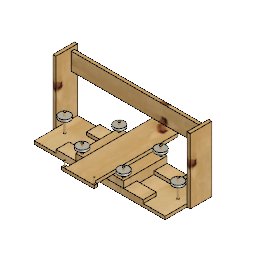
model_X v5 (Autodesk Fusion 360 design; units mm, degrees)
Autodesk Fusion 360 part; units mm, degrees
sketch "p1" plane through (0, 0, 0) normal (0, 0, 1) x (1, 0, 0)
  line L0 (300, 100) -> (-300, 100)
  line L1 (-300, 100) -> (-300, -100)
  line L2 (-300, -100) -> (300, -100)
  line L3 (300, -100) -> (300, 100)
  line L4 (300, 100) -> (-300, -100) construction
  line L5 (-300, 100) -> (300, -100) construction
  circle A0 centre (-260, 0) radius 5
  circle A1 centre (260, 0) radius 5
  line L6 (-200, -100) -> (200, -100)
  line L7 (200, -100) -> (200, -40)
  line L8 (200, -40) -> (-200, -40)
  line L9 (-200, -40) -> (-200, -100)
  line L10 (-200, 100) -> (200, 100)
  line L11 (200, 100) -> (200, 40)
  line L12 (200, 40) -> (-200, 40)
  line L13 (-200, 40) -> (-200, 100)
  circle A2 through (-235, 0, 75) (-272.5, 21.6506, 75) (-272.5, -21.6506, 75)
  circle A3 through (285, 0, 75) (247.5, 21.6506, 75) (247.5, -21.6506, 75)
  dimension "d1" = 600
  dimension "d2" = 200
  dimension "d3" = 40
  dimension "d4" = 40
  dimension "d5" = 10
  dimension "d6" = 10
  dimension "d7" = 400
  dimension "d8" = 60
  dimension "d9" = 400
  dimension "d10" = 60
  dimension "d11" = 100
  dimension "d12" = 100
  measures "d5" diameter of A0
  measures "d6" diameter of A1
  measures "d9" distance of L11 L13
  measures "d10" distance of L0 L12
  measures "d12" distance of L3 L7
extrude "Extrude1" add sketch "p1" along normal blind 15 contours L0 L1 L2 L3 L7 L8 L9 L11 L12 L13 | L0 L10 L11 L12 L13 | L2 L6 L7 L8 L9 | A0 | A1 makes body 1
extrude "Extrude2" add sketch "p1" along normal blind 30 contours L0 L10 L11 L12 L13 | L2 L6 L7 L8 L9 bodies 1
extrude "Extrude3" add sketch "p1" along normal blind 100 contours A0 | A1 bodies 1
ref_plane "WorkPlane1" through (0, 0, 30) normal (0, 0, 1) x (1, 0, 0)
sketch "p2" plane through (0, 0, 30) normal (0, 0, 1) x (1, 0, 0)
  line L0 (110, 39.5) -> (-110, 39.5)
  line L1 (-110, 39.5) -> (-110, -39.5)
  line L2 (-110, -39.5) -> (110, -39.5)
  line L3 (110, -39.5) -> (110, 39.5)
  line L4 (110, 39.5) -> (-110, -39.5) construction
  line L5 (-110, 39.5) -> (110, -39.5) construction
  line L6 (-110, 100) -> (110, 100)
  line L7 (110, 100) -> (110, -100)
  line L8 (110, -100) -> (-110, -100)
  line L9 (-110, -100) -> (-110, 100)
  line L10 (300, 100) -> (-300, 100)
  line L11 (-300, -100) -> (300, -100)
  circle A0 centre (-95, -85) radius 5
  circle A1 centre (95, -85) radius 5
  circle A2 centre (-95, 85) radius 5
  circle A3 centre (95, 85) radius 5
  circle A4 through (120, -85, 50) (82.5, -63.3494, 50) (82.5, -106.6506, 50)
  circle A5 through (-70, -85, 50) (-107.5, -63.3494, 50) (-107.5, -106.6506, 50)
  circle A6 through (-70, 85, 50) (-107.5, 106.6506, 50) (-107.5, 63.3494, 50)
  circle A7 through (120, 85, 50) (82.5, 106.6506, 50) (82.5, 63.3494, 50)
  line L12 (-70, -85) -> (-70, -100) construction
  line L13 (69.9377, -85) -> (70, -100) construction
  line L14 (70, 85) -> (70, 100) construction
  line L15 (-70, 85) -> (-70, 100) construction
  line L16 (70, -100) -> (60, -100) construction
  line L17 (-70, 100) -> (-60, 100) construction
  line L18 (-60, 100) -> (60, 100)
  line L19 (60, 100) -> (60, -100)
  line L20 (60, -100) -> (-60, -100)
  line L21 (-60, -100) -> (-60, 100)
  line L22 (30, 100) -> (-30, 100)
  line L23 (-30, 100) -> (-30, -100)
  line L24 (-30, -100) -> (30, -100)
  line L25 (30, -100) -> (30, 100)
  line L26 (30, 100) -> (-30, -100) construction
  line L27 (-30, 100) -> (30, -100) construction
  dimension "d20" = 220
  dimension "d21" = 79
  dimension "d22" = 220
  dimension "d27" = 10
  dimension "d28" = 15
  dimension "d29" = 15
  dimension "d30" = 10
  dimension "d31" = 10
  dimension "d32" = 10
  dimension "d33" = 15
  dimension "d34" = 15
  dimension "d35" = 15
  dimension "d36" = 15
  dimension "d37" = 15
  dimension "d38" = 15
  dimension "d59" = 10
  dimension "d60" = 10
  dimension "d61" = 120
  dimension "d62" = 200
  dimension "d63" = 60
  measures "d22" distance of L7 L9
  measures "d27" diameter of A0
  measures "d30" diameter of A1
  measures "d31" diameter of A2
  measures "d32" diameter of A3
extrude "Extrude6" add sketch "p2" against normal blind 14 separate body contours L0 L2 L3 L7 L19 | L0 L2 L19 L25 | L0 L2 L23 L25 | L0 L2 L21 L23 | L0 L1 L2 L9 L21 makes body 2
sketch "p1 (curves 75 mm off its plane)" plane through (0, 0, 75) normal (0, 0, 1) x (1, 0, 0)
  circle A0 centre (-260, 0) radius 25
  circle A1 centre (260, 0) radius 25
extrude "Extrude4" add sketch "p1 (curves 75 mm off its plane)" along normal blind 10 separate body makes body 3 at (-264.7538, 2.2158, 75) makes body 4 at (265.8316, 4.4538, 75)
extrude "Extrude7" add sketch "p2" along normal blind 15 contours L0 L2 L3 L7 L19 | L0 L6 L7 L10 L19 | L0 L2 L19 L25 | L0 L6 L10 L18 L19 L25 | L2 L7 L8 L11 L19 | L0 L2 L23 L25 | L0 L6 L10 L18 L22 L23 L25 | L2 L8 L11 L19 L20 L25 | L0 L2 L21 L23 | L0 L6 L10 L18 L21 L23 | L2 L8 L11 L20 L23 L24 L25 | L0 L1 L2 L9 L21 | L0 L6 L9 L10 L21 | L2 L8 L11 L20 L21 L23 | L2 L8 L9 L11 L21 | A0 | A1 | A2 | A3 bodies 2
extrude "Extrude8" add sketch "p2" along normal blind 70 contours A0 | A1 | A2 | A3 bodies 2
sketch "p2 (curves 50 mm off its plane)" plane through (0, 0, 80) normal (0, 0, 1) x (1, 0, 0)
  circle A0 centre (95, -85) radius 25
  circle A1 centre (-95, -85) radius 25
  circle A2 centre (-95, 85) radius 25
  circle A3 centre (95, 85) radius 25
extrude "Extrude9" add sketch "p2 (curves 50 mm off its plane)" along normal blind 10 separate body makes body 5 at (92.4105, -86.6853, 80) makes body 6 at (88.6141, 88.0753, 80) makes body 7 at (-97.5895, -86.6853, 80) makes body 8 at (-101.3859, 88.0753, 80)
extrude "Extrude10" add sketch "p2" along normal blind 30 contours L0 L2 L3 L7 L19 | L0 L6 L7 L10 L19 | L0 L2 L19 L25 | L0 L6 L10 L18 L19 L25 | L2 L7 L8 L11 L19 | L2 L8 L11 L19 L20 L25 | L0 L2 L21 L23 | L0 L6 L10 L18 L21 L23 | L0 L1 L2 L9 L21 | L0 L6 L9 L10 L21 | L2 L8 L11 L20 L21 L23 | L2 L8 L9 L11 L21 bodies 2
ref_plane "WorkPlane2" through (0, 0, 60) normal (0, 0, 1) x (1, 0, 0)
sketch "p3" plane through (0, 0, 60) normal (0, 0, 1) x (1, 0, 0)
  line L0 (-30, -100) -> (30, -100)
  line L1 (30, -100) -> (30, 100)
  line L2 (30, 100) -> (-30, 100)
  line L3 (-30, 100) -> (-30, -100)
  line L4 (60, 200) -> (-60, 200)
  line L5 (-60, 200) -> (-60, -200)
  line L6 (-60, -200) -> (60, -200)
  line L7 (60, -200) -> (60, 200)
  line L8 (60, 200) -> (-60, -200) construction
  line L9 (-60, 200) -> (60, -200) construction
  line L10 (60, -200) -> (75, -200)
  line L11 (75, -200) -> (75, -185)
  line L12 (75, -185) -> (60, -185)
  line L13 (60, -185) -> (60, -200)
  line L14 (-60, -200) -> (-75, -200)
  line L15 (-75, -200) -> (-75, -185)
  line L16 (-75, -185) -> (-60, -185)
  line L17 (-60, -185) -> (-60, -200)
  line L18 (-60, 200) -> (-75, 200)
  line L19 (-60, 185) -> (-60, 200)
  line L20 (60, 185) -> (60, 200)
  line L21 (10, 255) -> (-5, 255)
  line L22 (0, 200) -> (7.5, 200)
  line L23 (7.5, 200) -> (7.5, 240)
  line L24 (7.5, 240) -> (-7.5, 240)
  line L25 (-7.5, 240) -> (-7.5, 200)
  line L26 (7.5, 200) -> (-7.5, 200)
  circle A0 centre (0, 234.9202) radius 5
  circle A1 through (25, 234.9202, 20) (-12.5, 256.5708, 20) (-12.5, 213.2695, 20)
  circle A2 centre (-95, -85) radius 25 construction
  circle A3 centre (95, -85) radius 25 construction
  line L27 (-95, -110) -> (95, -110) construction
  line L28 (60, -100) -> (-60, -100) construction
  line L29 (-95, 110) -> (95, 110) construction
  circle A4 centre (67.5, -192.5) radius 2.5
  circle A5 centre (-67.5, -192.5) radius 2.5
  dimension "d67" = 400
  dimension "d72" = 15
  dimension "d73" = 15
  dimension "d74" = 15
  dimension "d75" = 15
  dimension "d82" = 7.5
  dimension "d83" = 40
  dimension "d84" = 15
  dimension "d87" = 10
  dimension "d93" = 220
  dimension "d94" = 90
  dimension "d95" = 90
  dimension "d96" = 5
  dimension "d97" = 5
  measures "d82" distance of origin
  measures "d87" diameter of A0
  measures "d94" distance of L4 L29
  measures "d95" distance of L10 L27
  measures "d96" diameter of A4
  measures "d97" diameter of A5
extrude "Extrude11" add sketch "p3" against normal blind 14 separate body contours L0 L1 L2 L3 makes body 9
extrude "Extrude12" add sketch "p3" along normal blind 15 contours L0 L1 L2 L3 | L4 L5 L6 L7 L13 L17 L19 L20 L22 L26 bodies 9
extrude "Extrude13" add sketch "p3" along normal blind 15 contours L4 L22 L23 L24 L25 L26 | L7 L10 L11 L12 L13 | L5 L14 L15 L16 L17 | A0 | A4 | A5 bodies 9
extrude "Extrude14" add sketch "p3" along normal blind 40 contours A0 bodies 9
sketch "p3 (curves 20 mm off its plane)" plane through (0, 0, 80) normal (0, 0, 1) x (1, 0, 0)
  circle A0 centre (0, 234.9202) radius 25
extrude "Extrude15" add sketch "p3 (curves 20 mm off its plane)" along normal blind 10 separate body makes body 10
copy_body "Body->Comp1" bodies 1 removing the originals makes body 11 in component "Component"
copy_body "Body->Comp2" bodies 2 removing the originals makes body 12 in component "Component'"
copy_body "Body->Comp3" bodies 9 removing the originals makes body 13 in component "Component''"
copy_body "CutPasteBodies1" bodies 10 removing the originals makes body 14 in component "Component''"
copy_body "CutPasteBodies1'" bodies 5 7 6 8 removing the originals makes body 15 makes body 16 makes body 17 makes body 18 in component "Component'"
copy_body "CutPasteBodies1''" bodies 4 3 removing the originals makes body 19 makes body 20 in component "Component"
extrude "Extrude1'" add sketch "p3" along normal blind 40 contours A4 | A5 bodies 13 in component "Component''"
sketch "linha" plane through (0.0019, 0.0411, 85) normal (0, 0, 1) x (-1, 0, 0)
  circle A0 centre (-259.9981, 0.0411) radius 25
  line L0 (-74.9981, 185.0411) -> (-59.9981, 185.0411)
  line L1 (-67.4981, 185.0411) -> (-69.9357, 85.0411)
  circle A1 centre (-94.9981, 85.0411) radius 25
  line L2 (-92.9821, 60.1225) -> (-261.4996, 24.996)
  circle A2 centre (-94.9981, -84.9589) radius 25
  line L3 (-262.0665, -24.8732) -> (-89.9342, -60.4771)
  circle A3 centre (0.0019, -234.8791) radius 25
  line L4 (-70.1205, -82.4879) -> (-59.9981, -199.9589)
  line L5 (-59.9981, -199.9589) -> (-20.3331, -249.4217)
  line L6 (22.409, -245.966) -> (60.0019, -199.9589)
  line L7 (60.0019, -199.9589) -> (70.0019, -84.9589)
  circle A4 centre (260.0019, 0.0411) radius 25
  circle A5 centre (95.0019, -84.9589) radius 25
  line L8 (260.8771, -24.9436) -> (89.9139, -60.4821)
  circle A6 centre (95.0019, 85.0411) radius 25
  line L9 (264.1198, 24.6996) -> (89.9608, 60.5546)
  line L10 (75.0019, 185.0411) -> (60.0019, 185.0411)
  line L11 (67.5019, 185.0411) -> (70.0019, 85.0411)
  arc A7 (70.0019, 85.0411) -> (89.9608, 60.5546) centre (95.0019, 85.0411) ccw
  arc A8 (-92.9821, 60.1225) -> (-69.9357, 85.0411) centre (-95.0512, 85.1528) ccw
  arc A9 (-261.4996, 24.996) -> (-262.0665, -24.8732) centre (-259.9981, 0.0411) ccw
  arc A10 (-69.9981, -84.9589) -> (-89.9342, -60.4771) centre (-94.9981, -84.9589) ccw
  arc A11 (-20.3331, -249.4217) -> (22.409, -245.966) centre (0.0019, -234.8791) ccw
  arc A12 (89.9139, -60.4821) -> (70.0019, -84.9589) centre (91.4397, -82.061) ccw
  arc A13 (260.8771, -24.9436) -> (264.1198, 24.6996) centre (260.0019, 0.0411) ccw
  line L12 (-67.4981, 185.0411) -> (-67.4981, 192)
  line L13 (67.5019, 185.0411) -> (67.5019, 190.4198)
  line L14 (67.5019, 190.4198) -> (67.5019, 192)
sketch "Sketch5" plane through (0, 0, 0) normal (0, 0, 1) x (1, 0, 0)
  line L0 (300, 0) -> (315, 0)
  line L1 (315, 0) -> (315, 100)
  line L2 (315, 100) -> (300, 100)
  line L3 (300, 100) -> (300, 0)
  line L4 (300, -100) -> (300, 100)
  line L5 (-300, 0) -> (-315, 0)
  line L6 (-315, 0) -> (-315, 100)
  line L7 (-315, 100) -> (-300, 100)
  line L8 (-300, 100) -> (-300, 0)
  dimension "d100" = 15
  dimension "d101" = 15
extrude "Extrude16" add sketch "Sketch5" along normal blind 300 separate body makes body 21 at (300, 66.6667, 100) makes body 22 at (-315, 33.3333, 100)
sketch "Sketch6" plane through (300, 0, 0) normal (-1, 0, 0) x (0, -1, 0)
  line L0 (-100, 0) -> (0, 0)
  line L1 (0, 0) -> (0, 300)
  line L2 (0, 300) -> (-100, 300)
  line L3 (-100, 300) -> (-100, 0)
  line L4 (-85, 205) -> (-70, 205)
  line L5 (-70, 205) -> (-70, 285)
  line L6 (-70, 285) -> (-85, 285)
  line L7 (-85, 285) -> (-85, 205)
extrude "Extrude17" add sketch "Sketch6" along normal blind 600 contours L4 L5 L6 L7 bodies 21 22
copy_body "Body->Comp4" bodies 21 removing the originals makes body 23 in component "Component'''"
component "Component" placed x (1, 0, 0) y (0, 1, 0) z (0, 0, 1) at (0, 0, 0)
component "Component'" placed x (1, 0, 0) y (0, 1, 0) z (0, 0, 1) at (0, 0, 0)
component "Component''" placed x (1, 0, 0) y (0, 1, 0) z (0, 0, 1) at (0, 0, 0)
component "Component'''" placed x (1, 0, 0) y (0, 1, 0) z (0, 0, 1) at (0, 0, 0)
equation "d4 = d3"
equation "d6 = d5"
equation "d9 = d7"
equation "d10 = d8"
equation "d12 = d11"
equation "d22 = d20"
equation "d33 = d29"
equation "d34 = d28"
equation "d35 = d29"
equation "d36 = d28"
equation "d37 = d29"
equation "d38 = d28"
named bodies: "rolamento1", "rolamento2", "rolamento3", "rolamento4", "rolamento5", "rolamento6"
